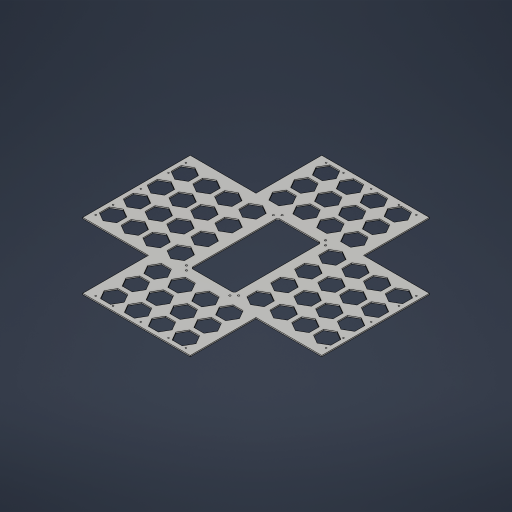
# Autodesk Inventor part: 200510
Saved by Autodesk Inventor 2023 (Build 270158000, 158)
## iProperties
Created: 2022-08-10
Part Number: 200510
Material: Aluminum 5052 H32
Document SubType Name: Sheet Metal
Designer: robotics
Density: 2.7 g/cm^3
Sheet Metal Rule: .125 5052
Appearance: Aluminum - Flat
Mass: 1564.52 g
Surface Area: 4087.8 cm^2
Volume: 579.451 cm^3
Description: Baseplate with concept geometry for pdp riser
GlobalPropertyList: <PropertyList/>
DocNumber: 200510updated.ipt
Folder: .
VDS_Category: CAD
Author: robotics
Autodesk Inventor part; units mm, degrees
ref_plane "YZ Plane" through (0, 0, 0) normal (1, 0, 0) x (0, 1, 0)
ref_plane "XZ Plane" through (0, 0, 0) normal (0, 1, 0) x (-1, 0, 0)
ref_plane "XY Plane" through (0, 0, 0) normal (0, 0, 1) x (1, 0, 0)
sketch "Sketch1" plane through (0, 0, 0) normal (0, 1, 0) x (-1, 0, 0)
  line L0 (0, 0) -> (0, -314.325)
  line L1 (0, -314.325) -> (192.0875, -314.325)
  line L2 (192.0875, -314.325) -> (192.0875, -506.4125)
  line L3 (192.0875, -506.4125) -> (506.4125, -506.4125)
  line L4 (506.4125, -506.4125) -> (506.4125, -314.325)
  line L5 (506.4125, -314.325) -> (698.5, -314.325)
  line L6 (698.5, -314.325) -> (698.5, 0)
  line L7 (698.5, 0) -> (506.4125, 0)
  line L8 (506.4125, 0) -> (506.4125, 192.0875)
  line L9 (506.4125, 192.0875) -> (192.0875, 192.0875)
  line L10 (192.0875, 192.0875) -> (192.0875, 0)
  line L11 (192.0875, 0) -> (0, 0)
  line L12 (698.5, 192.0875) -> (0, 192.0875) construction
  line L13 (0, 192.0875) -> (0, -506.4125) construction
  line L14 (0, -506.4125) -> (698.5, -506.4125) construction
  line L15 (698.5, -506.4125) -> (698.5, 192.0875) construction
  line L16 (0, -157.1625) -> (698.5, -157.1625) construction
  line L17 (349.25, 192.0875) -> (349.25, -506.4125) construction
  line L18 (412.75, -284.1625) -> (285.75, -284.1625)
  line L19 (285.75, -284.1625) -> (285.75, -30.1625)
  line L20 (285.75, -30.1625) -> (412.75, -30.1625)
  line L21 (412.75, -30.1625) -> (412.75, -284.1625)
  line L22 (412.75, -284.1625) -> (285.75, -30.1625) construction
  line L23 (285.75, -284.1625) -> (412.75, -30.1625) construction
  line L24 (285.75, -30.1625) -> (273.05, -30.1625) construction
  line L25 (285.75, -30.1625) -> (285.75, -17.4625) construction
  line L26 (412.75, -30.1625) -> (425.45, -30.1625) construction
  line L27 (412.75, -30.1625) -> (412.75, -17.4625) construction
  line L28 (412.75, -284.1625) -> (425.45, -284.1625) construction
  line L29 (412.75, -284.1625) -> (412.75, -296.8625) construction
  line L30 (285.75, -284.1625) -> (273.05, -284.1625) construction
  line L31 (285.75, -284.1625) -> (285.75, -296.8625) construction
  circle A0 centre (425.45, -30.1625) radius 2.5797
  circle A1 centre (412.75, -17.4625) radius 2.5797
  circle A2 centre (285.75, -17.4625) radius 2.5797
  circle A3 centre (273.05, -30.1625) radius 2.5797
  circle A4 centre (273.05, -284.1625) radius 2.5797
  circle A5 centre (285.75, -296.8625) radius 2.5797
  circle A6 centre (412.75, -296.8625) radius 2.5797
  circle A7 centre (425.45, -284.1625) radius 2.5797
  line L32 (213.5581, 153.9875) -> (228.2228, 179.3875)
  line L33 (228.2228, 179.3875) -> (257.5522, 179.3875)
  line L34 (257.5522, 179.3875) -> (272.2169, 153.9875)
  line L35 (272.2169, 153.9875) -> (257.5522, 128.5875)
  line L36 (257.5522, 128.5875) -> (228.2228, 128.5875)
  line L37 (228.2228, 128.5875) -> (213.5581, 153.9875)
  line L38 (298.0728, 179.3875) -> (327.4022, 179.3875)
  line L39 (283.4081, 153.9875) -> (298.0728, 179.3875)
  line L40 (298.0728, 128.5875) -> (283.4081, 153.9875)
  line L41 (327.4022, 128.5875) -> (298.0728, 128.5875)
  line L42 (342.0669, 153.9875) -> (327.4022, 128.5875)
  line L43 (327.4022, 179.3875) -> (342.0669, 153.9875)
  line L44 (367.9228, 179.3875) -> (397.2522, 179.3875)
  line L45 (353.2581, 153.9875) -> (367.9228, 179.3875)
  line L46 (367.9228, 128.5875) -> (353.2581, 153.9875)
  line L47 (397.2522, 128.5875) -> (367.9228, 128.5875)
  line L48 (411.9169, 153.9875) -> (397.2522, 128.5875)
  line L49 (397.2522, 179.3875) -> (411.9169, 153.9875)
  line L50 (437.7728, 179.3875) -> (467.1022, 179.3875)
  line L51 (423.1081, 153.9875) -> (437.7728, 179.3875)
  line L52 (437.7728, 128.5875) -> (423.1081, 153.9875)
  line L53 (467.1022, 128.5875) -> (437.7728, 128.5875)
  line L54 (481.7669, 153.9875) -> (467.1022, 128.5875)
  line L55 (467.1022, 179.3875) -> (481.7669, 153.9875)
  line L56 (228.2228, 115.8875) -> (257.5522, 115.8875)
  line L57 (213.5581, 90.4875) -> (228.2228, 115.8875)
  line L58 (228.2228, 65.0875) -> (213.5581, 90.4875)
  line L59 (257.5522, 65.0875) -> (228.2228, 65.0875)
  line L60 (272.2169, 90.4875) -> (257.5522, 65.0875)
  line L61 (257.5522, 115.8875) -> (272.2169, 90.4875)
  line L62 (298.0728, 115.8875) -> (327.4022, 115.8875)
  line L63 (283.4081, 90.4875) -> (298.0728, 115.8875)
  line L64 (298.0728, 65.0875) -> (283.4081, 90.4875)
  line L65 (327.4022, 65.0875) -> (298.0728, 65.0875)
  line L66 (342.0669, 90.4875) -> (327.4022, 65.0875)
  line L67 (327.4022, 115.8875) -> (342.0669, 90.4875)
  line L68 (367.9228, 115.8875) -> (397.2522, 115.8875)
  line L69 (353.2581, 90.4875) -> (367.9228, 115.8875)
  line L70 (367.9228, 65.0875) -> (353.2581, 90.4875)
  line L71 (397.2522, 65.0875) -> (367.9228, 65.0875)
  line L72 (411.9169, 90.4875) -> (397.2522, 65.0875)
  line L73 (397.2522, 115.8875) -> (411.9169, 90.4875)
  line L74 (437.7728, 115.8875) -> (467.1022, 115.8875)
  line L75 (423.1081, 90.4875) -> (437.7728, 115.8875)
  line L76 (437.7728, 65.0875) -> (423.1081, 90.4875)
  line L77 (467.1022, 65.0875) -> (437.7728, 65.0875)
  line L78 (481.7669, 90.4875) -> (467.1022, 65.0875)
  line L79 (467.1022, 115.8875) -> (481.7669, 90.4875)
  line L80 (228.2228, 52.3875) -> (257.5522, 52.3875)
  line L81 (213.5581, 26.9875) -> (228.2228, 52.3875)
  line L82 (228.2228, 1.5875) -> (213.5581, 26.9875)
  line L83 (257.5522, 1.5875) -> (228.2228, 1.5875)
  line L84 (272.2169, 26.9875) -> (257.5522, 1.5875)
  line L85 (257.5522, 52.3875) -> (272.2169, 26.9875)
  line L86 (298.0728, 52.3875) -> (327.4022, 52.3875)
  line L87 (283.4081, 26.9875) -> (298.0728, 52.3875)
  line L88 (298.0728, 1.5875) -> (283.4081, 26.9875)
  line L89 (327.4022, 1.5875) -> (298.0728, 1.5875)
  line L90 (342.0669, 26.9875) -> (327.4022, 1.5875)
  line L91 (327.4022, 52.3875) -> (342.0669, 26.9875)
  line L92 (367.9228, 52.3875) -> (397.2522, 52.3875)
  line L93 (353.2581, 26.9875) -> (367.9228, 52.3875)
  line L94 (367.9228, 1.5875) -> (353.2581, 26.9875)
  line L95 (397.2522, 1.5875) -> (367.9228, 1.5875)
  line L96 (411.9169, 26.9875) -> (397.2522, 1.5875)
  line L97 (397.2522, 52.3875) -> (411.9169, 26.9875)
  line L98 (437.7728, 52.3875) -> (467.1022, 52.3875)
  line L99 (423.1081, 26.9875) -> (437.7728, 52.3875)
  line L100 (437.7728, 1.5875) -> (423.1081, 26.9875)
  line L101 (467.1022, 1.5875) -> (437.7728, 1.5875)
  line L102 (481.7669, 26.9875) -> (467.1022, 1.5875)
  line L103 (467.1022, 52.3875) -> (481.7669, 26.9875)
  line L104 (38.1, -292.8544) -> (12.7, -278.1897)
  line L105 (12.7, -278.1897) -> (12.7, -248.8603)
  line L106 (12.7, -248.8603) -> (38.1, -234.1956)
  line L107 (38.1, -234.1956) -> (63.5, -248.8603)
  line L108 (127, -278.1897) -> (101.6, -292.8544)
  line L109 (101.6, -234.1956) -> (127, -248.8603)
  line L110 (76.2, -248.8603) -> (101.6, -234.1956)
  line L111 (76.2, -278.1897) -> (76.2, -248.8603)
  line L112 (101.6, -292.8544) -> (76.2, -278.1897)
  line L113 (63.5, -248.8603) -> (63.5, -278.1897)
  line L114 (63.5, -278.1897) -> (38.1, -292.8544)
  line L115 (127, -248.8603) -> (127, -278.1897)
  line L116 (12.7, -208.3397) -> (12.7, -179.0103)
  line L117 (127, -208.3397) -> (101.6, -223.0044)
  line L118 (12.7, -138.4897) -> (12.7, -109.1603)
  line L119 (101.6, -223.0044) -> (76.2, -208.3397)
  line L120 (76.2, -208.3397) -> (76.2, -179.0103)
  line L121 (63.5, -138.4897) -> (38.1, -153.1544)
  line L122 (38.1, -153.1544) -> (12.7, -138.4897)
  line L123 (38.1, -164.3456) -> (63.5, -179.0103)
  line L124 (63.5, -179.0103) -> (63.5, -208.3397)
  line L125 (63.5, -208.3397) -> (38.1, -223.0044)
  line L126 (12.7, -179.0103) -> (38.1, -164.3456)
  line L127 (38.1, -223.0044) -> (12.7, -208.3397)
  line L128 (38.1, -94.4956) -> (63.5, -109.1603)
  line L129 (12.7, -109.1603) -> (38.1, -94.4956)
  line L130 (63.5, -39.3103) -> (63.5, -68.6397)
  line L131 (38.1, -24.6456) -> (63.5, -39.3103)
  line L132 (63.5, -68.6397) -> (38.1, -83.3044)
  line L133 (12.7, -39.3103) -> (38.1, -24.6456)
  line L134 (12.7, -68.6397) -> (12.7, -39.3103)
  line L135 (38.1, -83.3044) -> (12.7, -68.6397)
  line L136 (76.2, -179.0103) -> (101.6, -164.3456)
  line L137 (101.6, -164.3456) -> (127, -179.0103)
  line L138 (63.5, -109.1603) -> (63.5, -138.4897)
  line L139 (101.6, -153.1544) -> (76.2, -138.4897)
  line L140 (76.2, -138.4897) -> (76.2, -109.1603)
  line L141 (127, -138.4897) -> (101.6, -153.1544)
  line L142 (76.2, -68.6397) -> (76.2, -39.3103)
  line L143 (76.2, -109.1603) -> (101.6, -94.4956)
  line L144 (101.6, -83.3044) -> (76.2, -68.6397)
  line L145 (101.6, -94.4956) -> (127, -109.1603)
  line L146 (127, -68.6397) -> (101.6, -83.3044)
  line L147 (76.2, -39.3103) -> (101.6, -24.6456)
  line L148 (127, -39.3103) -> (127, -68.6397)
  line L149 (101.6, -24.6456) -> (127, -39.3103)
  line L150 (139.7, -278.1897) -> (139.7, -248.8603)
  line L151 (165.1, -292.8544) -> (139.7, -278.1897)
  line L152 (139.7, -248.8603) -> (165.1, -234.1956)
  line L153 (165.1, -223.0044) -> (139.7, -208.3397)
  line L154 (190.5, -278.1897) -> (165.1, -292.8544)
  line L155 (190.5, -248.8603) -> (190.5, -278.1897)
  line L156 (165.1, -234.1956) -> (190.5, -248.8603)
  line L157 (190.5, -208.3397) -> (165.1, -223.0044)
  line L158 (127, -179.0103) -> (127, -208.3397)
  line L159 (139.7, -208.3397) -> (139.7, -179.0103)
  line L160 (190.5, -179.0103) -> (190.5, -208.3397)
  line L161 (127, -109.1603) -> (127, -138.4897)
  line L162 (165.1, -153.1544) -> (139.7, -138.4897)
  line L163 (165.1, -164.3456) -> (190.5, -179.0103)
  line L164 (139.7, -138.4897) -> (139.7, -109.1603)
  line L165 (190.5, -138.4897) -> (165.1, -153.1544)
  line L166 (190.5, -109.1603) -> (190.5, -138.4897)
  line L167 (139.7, -179.0103) -> (165.1, -164.3456)
  line L168 (165.1, -94.4956) -> (190.5, -109.1603)
  line L169 (139.7, -109.1603) -> (165.1, -94.4956)
  line L170 (190.5, -68.6397) -> (165.1, -83.3044)
  line L171 (190.5, -39.3103) -> (190.5, -68.6397)
  line L172 (139.7, -68.6397) -> (139.7, -39.3103)
  line L173 (165.1, -24.6456) -> (190.5, -39.3103)
  line L174 (139.7, -39.3103) -> (165.1, -24.6456)
  line L175 (165.1, -83.3044) -> (139.7, -68.6397)
  line L176 (484.9419, -468.3125) -> (470.2772, -493.7125)
  line L177 (470.2772, -493.7125) -> (440.9478, -493.7125)
  line L178 (440.9478, -493.7125) -> (426.2831, -468.3125)
  line L179 (426.2831, -468.3125) -> (440.9478, -442.9125)
  line L180 (470.2772, -379.4125) -> (484.9419, -404.8125)
  line L181 (426.2831, -404.8125) -> (440.9478, -379.4125)
  line L182 (440.9478, -430.2125) -> (426.2831, -404.8125)
  line L183 (470.2772, -430.2125) -> (440.9478, -430.2125)
  line L184 (484.9419, -404.8125) -> (470.2772, -430.2125)
  line L185 (440.9478, -442.9125) -> (470.2772, -442.9125)
  line L186 (470.2772, -442.9125) -> (484.9419, -468.3125)
  line L187 (440.9478, -379.4125) -> (470.2772, -379.4125)
  line L188 (400.4272, -493.7125) -> (371.0978, -493.7125)
  line L189 (400.4272, -379.4125) -> (415.0919, -404.8125)
  line L190 (330.5772, -493.7125) -> (301.2478, -493.7125)
  line L191 (415.0919, -404.8125) -> (400.4272, -430.2125)
  line L192 (400.4272, -430.2125) -> (371.0978, -430.2125)
  line L193 (330.5772, -442.9125) -> (345.2419, -468.3125)
  line L194 (345.2419, -468.3125) -> (330.5772, -493.7125)
  line L195 (356.4331, -468.3125) -> (371.0978, -442.9125)
  line L196 (371.0978, -442.9125) -> (400.4272, -442.9125)
  line L197 (400.4272, -442.9125) -> (415.0919, -468.3125)
  line L198 (371.0978, -493.7125) -> (356.4331, -468.3125)
  line L199 (415.0919, -468.3125) -> (400.4272, -493.7125)
  line L200 (286.5831, -468.3125) -> (301.2478, -442.9125)
  line L201 (301.2478, -493.7125) -> (286.5831, -468.3125)
  line L202 (231.3978, -442.9125) -> (260.7272, -442.9125)
  line L203 (216.7331, -468.3125) -> (231.3978, -442.9125)
  line L204 (260.7272, -442.9125) -> (275.3919, -468.3125)
  line L205 (231.3978, -493.7125) -> (216.7331, -468.3125)
  line L206 (260.7272, -493.7125) -> (231.3978, -493.7125)
  line L207 (275.3919, -468.3125) -> (260.7272, -493.7125)
  line L208 (371.0978, -430.2125) -> (356.4331, -404.8125)
  line L209 (356.4331, -404.8125) -> (371.0978, -379.4125)
  line L210 (301.2478, -442.9125) -> (330.5772, -442.9125)
  line L211 (345.2419, -404.8125) -> (330.5772, -430.2125)
  line L212 (330.5772, -430.2125) -> (301.2478, -430.2125)
  line L213 (330.5772, -379.4125) -> (345.2419, -404.8125)
  line L214 (260.7272, -430.2125) -> (231.3978, -430.2125)
  line L215 (301.2478, -430.2125) -> (286.5831, -404.8125)
  line L216 (275.3919, -404.8125) -> (260.7272, -430.2125)
  line L217 (286.5831, -404.8125) -> (301.2478, -379.4125)
  line L218 (260.7272, -379.4125) -> (275.3919, -404.8125)
  line L219 (231.3978, -430.2125) -> (216.7331, -404.8125)
  line L220 (231.3978, -379.4125) -> (260.7272, -379.4125)
  line L221 (216.7331, -404.8125) -> (231.3978, -379.4125)
  line L222 (470.2772, -366.7125) -> (440.9478, -366.7125)
  line L223 (484.9419, -341.3125) -> (470.2772, -366.7125)
  line L224 (440.9478, -366.7125) -> (426.2831, -341.3125)
  line L225 (415.0919, -341.3125) -> (400.4272, -366.7125)
  line L226 (470.2772, -315.9125) -> (484.9419, -341.3125)
  line L227 (440.9478, -315.9125) -> (470.2772, -315.9125)
  line L228 (426.2831, -341.3125) -> (440.9478, -315.9125)
  line L229 (400.4272, -315.9125) -> (415.0919, -341.3125)
  line L230 (371.0978, -379.4125) -> (400.4272, -379.4125)
  line L231 (400.4272, -366.7125) -> (371.0978, -366.7125)
  line L232 (371.0978, -315.9125) -> (400.4272, -315.9125)
  line L233 (301.2478, -379.4125) -> (330.5772, -379.4125)
  line L234 (345.2419, -341.3125) -> (330.5772, -366.7125)
  line L235 (356.4331, -341.3125) -> (371.0978, -315.9125)
  line L236 (330.5772, -366.7125) -> (301.2478, -366.7125)
  line L237 (330.5772, -315.9125) -> (345.2419, -341.3125)
  line L238 (301.2478, -315.9125) -> (330.5772, -315.9125)
  line L239 (371.0978, -366.7125) -> (356.4331, -341.3125)
  line L240 (286.5831, -341.3125) -> (301.2478, -315.9125)
  line L241 (301.2478, -366.7125) -> (286.5831, -341.3125)
  line L242 (260.7272, -315.9125) -> (275.3919, -341.3125)
  line L243 (231.3978, -315.9125) -> (260.7272, -315.9125)
  line L244 (260.7272, -366.7125) -> (231.3978, -366.7125)
  line L245 (216.7331, -341.3125) -> (231.3978, -315.9125)
  line L246 (231.3978, -366.7125) -> (216.7331, -341.3125)
  line L247 (275.3919, -341.3125) -> (260.7272, -366.7125)
  line L248 (660.4, -21.4706) -> (685.8, -36.1353)
  line L249 (685.8, -36.1353) -> (685.8, -65.4647)
  line L250 (685.8, -65.4647) -> (660.4, -80.1294)
  line L251 (660.4, -80.1294) -> (635, -65.4647)
  line L252 (571.5, -36.1353) -> (596.9, -21.4706)
  line L253 (596.9, -80.1294) -> (571.5, -65.4647)
  line L254 (622.3, -65.4647) -> (596.9, -80.1294)
  line L255 (622.3, -36.1353) -> (622.3, -65.4647)
  line L256 (596.9, -21.4706) -> (622.3, -36.1353)
  line L257 (635, -65.4647) -> (635, -36.1353)
  line L258 (635, -36.1353) -> (660.4, -21.4706)
  line L259 (571.5, -65.4647) -> (571.5, -36.1353)
  line L260 (685.8, -105.9853) -> (685.8, -135.3147)
  line L261 (571.5, -105.9853) -> (596.9, -91.3206)
  line L262 (685.8, -175.8353) -> (685.8, -205.1647)
  line L263 (596.9, -91.3206) -> (622.3, -105.9853)
  line L264 (622.3, -105.9853) -> (622.3, -135.3147)
  line L265 (635, -175.8353) -> (660.4, -161.1706)
  line L266 (660.4, -161.1706) -> (685.8, -175.8353)
  line L267 (660.4, -149.9794) -> (635, -135.3147)
  line L268 (635, -135.3147) -> (635, -105.9853)
  line L269 (635, -105.9853) -> (660.4, -91.3206)
  line L270 (685.8, -135.3147) -> (660.4, -149.9794)
  line L271 (660.4, -91.3206) -> (685.8, -105.9853)
  line L272 (660.4, -219.8294) -> (635, -205.1647)
  line L273 (685.8, -205.1647) -> (660.4, -219.8294)
  line L274 (635, -275.0147) -> (635, -245.6853)
  line L275 (660.4, -289.6794) -> (635, -275.0147)
  line L276 (635, -245.6853) -> (660.4, -231.0206)
  line L277 (685.8, -275.0147) -> (660.4, -289.6794)
  line L278 (685.8, -245.6853) -> (685.8, -275.0147)
  line L279 (660.4, -231.0206) -> (685.8, -245.6853)
  line L280 (622.3, -135.3147) -> (596.9, -149.9794)
  line L281 (596.9, -149.9794) -> (571.5, -135.3147)
  line L282 (635, -205.1647) -> (635, -175.8353)
  line L283 (596.9, -161.1706) -> (622.3, -175.8353)
  line L284 (622.3, -175.8353) -> (622.3, -205.1647)
  line L285 (571.5, -175.8353) -> (596.9, -161.1706)
  line L286 (622.3, -245.6853) -> (622.3, -275.0147)
  line L287 (622.3, -205.1647) -> (596.9, -219.8294)
  line L288 (596.9, -231.0206) -> (622.3, -245.6853)
  line L289 (596.9, -219.8294) -> (571.5, -205.1647)
  line L290 (571.5, -245.6853) -> (596.9, -231.0206)
  line L291 (622.3, -275.0147) -> (596.9, -289.6794)
  line L292 (571.5, -275.0147) -> (571.5, -245.6853)
  line L293 (596.9, -289.6794) -> (571.5, -275.0147)
  line L294 (558.8, -36.1353) -> (558.8, -65.4647)
  line L295 (533.4, -21.4706) -> (558.8, -36.1353)
  line L296 (558.8, -65.4647) -> (533.4, -80.1294)
  line L297 (533.4, -91.3206) -> (558.8, -105.9853)
  line L298 (508, -36.1353) -> (533.4, -21.4706)
  line L299 (508, -65.4647) -> (508, -36.1353)
  line L300 (533.4, -80.1294) -> (508, -65.4647)
  line L301 (508, -105.9853) -> (533.4, -91.3206)
  line L302 (571.5, -135.3147) -> (571.5, -105.9853)
  line L303 (558.8, -105.9853) -> (558.8, -135.3147)
  line L304 (508, -135.3147) -> (508, -105.9853)
  line L305 (571.5, -205.1647) -> (571.5, -175.8353)
  line L306 (533.4, -161.1706) -> (558.8, -175.8353)
  line L307 (533.4, -149.9794) -> (508, -135.3147)
  line L308 (558.8, -175.8353) -> (558.8, -205.1647)
  line L309 (508, -175.8353) -> (533.4, -161.1706)
  line L310 (508, -205.1647) -> (508, -175.8353)
  line L311 (558.8, -135.3147) -> (533.4, -149.9794)
  line L312 (533.4, -219.8294) -> (508, -205.1647)
  line L313 (558.8, -205.1647) -> (533.4, -219.8294)
  line L314 (508, -245.6853) -> (533.4, -231.0206)
  line L315 (508, -275.0147) -> (508, -245.6853)
  line L316 (558.8, -245.6853) -> (558.8, -275.0147)
  line L317 (533.4, -289.6794) -> (508, -275.0147)
  line L318 (558.8, -275.0147) -> (533.4, -289.6794)
  line L319 (533.4, -231.0206) -> (558.8, -245.6853)
  line L320 (258.0906, -39.3103) -> (258.0906, -68.6397)
  line L321 (258.0906, -68.6397) -> (232.6906, -83.3044)
  line L322 (232.6906, -83.3044) -> (207.2906, -68.6397)
  line L323 (207.2906, -68.6397) -> (207.2906, -39.3103)
  line L324 (207.2906, -39.3103) -> (232.6906, -24.6456)
  line L325 (232.6906, -24.6456) -> (258.0906, -39.3103)
  line L326 (232.6906, -153.1544) -> (207.2906, -138.4897)
  line L327 (207.2906, -138.4897) -> (207.2906, -109.1603)
  line L328 (207.2906, -109.1603) -> (232.6906, -94.4956)
  line L329 (232.6906, -94.4956) -> (258.0906, -109.1603)
  line L330 (258.0906, -109.1603) -> (258.0906, -138.4897)
  line L331 (258.0906, -138.4897) -> (232.6906, -153.1544)
  line L332 (232.6906, -223.0044) -> (207.2906, -208.3397)
  line L333 (207.2906, -208.3397) -> (207.2906, -179.0103)
  line L334 (207.2906, -179.0103) -> (232.6906, -164.3456)
  line L335 (232.6906, -164.3456) -> (258.0906, -179.0103)
  line L336 (258.0906, -179.0103) -> (258.0906, -208.3397)
  line L337 (258.0906, -208.3397) -> (232.6906, -223.0044)
  line L338 (232.6906, -292.8544) -> (207.2906, -278.1897)
  line L339 (207.2906, -278.1897) -> (207.2906, -248.8603)
  line L340 (207.2906, -248.8603) -> (232.6906, -234.1956)
  line L341 (232.6906, -234.1956) -> (258.0906, -248.8603)
  line L342 (258.0906, -248.8603) -> (258.0906, -278.1897)
  line L343 (258.0906, -278.1897) -> (232.6906, -292.8544)
  line L344 (440.4094, -39.3103) -> (440.4094, -68.6397)
  line L345 (440.4094, -68.6397) -> (465.8094, -83.3044)
  line L346 (465.8094, -83.3044) -> (491.2094, -68.6397)
  line L347 (491.2094, -68.6397) -> (491.2094, -39.3103)
  line L348 (491.2094, -39.3103) -> (465.8094, -24.6456)
  line L349 (465.8094, -24.6456) -> (440.4094, -39.3103)
  line L350 (465.8094, -153.1544) -> (491.2094, -138.4897)
  line L351 (491.2094, -138.4897) -> (491.2094, -109.1603)
  line L352 (491.2094, -109.1603) -> (465.8094, -94.4956)
  line L353 (465.8094, -94.4956) -> (440.4094, -109.1603)
  line L354 (440.4094, -109.1603) -> (440.4094, -138.4897)
  line L355 (440.4094, -138.4897) -> (465.8094, -153.1544)
  line L356 (465.8094, -223.0044) -> (491.2094, -208.3397)
  line L357 (491.2094, -208.3397) -> (491.2094, -179.0103)
  line L358 (491.2094, -179.0103) -> (465.8094, -164.3456)
  line L359 (465.8094, -164.3456) -> (440.4094, -179.0103)
  line L360 (440.4094, -179.0103) -> (440.4094, -208.3397)
  line L361 (440.4094, -208.3397) -> (465.8094, -223.0044)
  line L362 (465.8094, -292.8544) -> (491.2094, -278.1897)
  line L363 (491.2094, -278.1897) -> (491.2094, -248.8603)
  line L364 (491.2094, -248.8603) -> (465.8094, -234.1956)
  line L365 (465.8094, -234.1956) -> (440.4094, -248.8603)
  line L366 (440.4094, -248.8603) -> (440.4094, -278.1897)
  line L367 (440.4094, -278.1897) -> (465.8094, -292.8544)
  point P0 (349.25, -157.1625)
  point P1 (242.8875, 153.9875)
  point P2 (312.7375, 153.9875)
  point P3 (382.5875, 153.9875)
  point P4 (452.4375, 153.9875)
  point P5 (242.8875, 90.4875)
  point P6 (312.7375, 90.4875)
  point P7 (382.5875, 90.4875)
  point P8 (452.4375, 90.4875)
  point P9 (242.8875, 26.9875)
  point P10 (312.7375, 26.9875)
  point P11 (382.5875, 26.9875)
  point P12 (452.4375, 26.9875)
  point P13 (38.1, -263.525)
  point P14 (101.6, -263.525)
  point P15 (101.6, -193.675)
  point P16 (38.1, -193.675)
  point P17 (38.1, -53.975)
  point P18 (38.1, -123.825)
  point P19 (101.6, -123.825)
  point P20 (101.6, -53.975)
  point P21 (165.1, -263.525)
  point P22 (165.1, -193.675)
  point P23 (165.1, -123.825)
  point P24 (165.1, -53.975)
  point P25 (455.6125, -468.3125)
  point P26 (455.6125, -404.8125)
  point P27 (385.7625, -404.8125)
  point P28 (385.7625, -468.3125)
  point P29 (246.0625, -468.3125)
  point P30 (315.9125, -468.3125)
  point P31 (315.9125, -404.8125)
  point P32 (246.0625, -404.8125)
  point P33 (455.6125, -341.3125)
  point P34 (385.7625, -341.3125)
  point P35 (315.9125, -341.3125)
  point P36 (246.0625, -341.3125)
  point P37 (660.4, -50.8)
  point P38 (596.9, -50.8)
  point P39 (596.9, -120.65)
  point P40 (660.4, -120.65)
  point P41 (660.4, -260.35)
  point P42 (660.4, -190.5)
  point P43 (596.9, -190.5)
  point P44 (596.9, -260.35)
  point P45 (533.4, -50.8)
  point P46 (533.4, -120.65)
  point P47 (533.4, -190.5)
  point P48 (533.4, -260.35)
  point P49 (232.6906, -53.975)
  point P50 (232.6906, -123.825)
  point P51 (232.6906, -193.675)
  point P52 (232.6906, -263.525)
  point P53 (465.8094, -53.975)
  point P54 (465.8094, -123.825)
  point P55 (465.8094, -193.675)
  point P56 (465.8094, -263.525)
  dimension "d0" = 698.5
  dimension "d1" = 192.0875
  dimension "d43" = 127
  dimension "d44" = 254
  dimension "d46" = 12.7
  dimension "d47" = 12.7
  dimension "d48" = 12.7
  dimension "d49" = 12.7
  dimension "d50" = 12.7
  dimension "d51" = 12.7
  dimension "d52" = 12.7
  dimension "d53" = 12.7
  dimension "d54" = 5.1594
  dimension "d55" = 25.4
  dimension "d56" = 38.1
  dimension "d57" = 50.8
  dimension "d60" = 69.85
  dimension "d63" = 63.5
  dimension "d68" = 360
  dimension "d72" = 69.85
  dimension "d77" = 16.7906
  measures "d0" distance of L14.end L12.start
  measures "d1" distance of L7.end L8.end
  measures "d43" distance of L19.end L20.end
  measures "d44" distance of L18.end L19.end
  measures "d46" distance of L19.end L24.end
  measures "d47" distance of L19.end L25.end
  measures "d48" distance of L20.end L26.end
  measures "d49" distance of L20.end L27.end
  measures "d50" distance of L18.start L28.end
  measures "d51" distance of L18.start L29.end
  measures "d52" distance of L18.end L30.end
  measures "d53" distance of L18.end L31.end
  measures "d54" diameter of A0
  measures "d55" vertical distance of L33.end L34.end
  measures "d56" distance from line of L9 point (242.887, 153.988)
  measures "d57" distance from line of L10 point (242.887, 153.988)
  measures "d60" distance of L32.end L38.start
  measures "d63" distance of L32.end L56.start
  measures "d72" distance of point (232.691, -53.975) point (232.691, -123.825)
  measures "d77" distance between parallel lines of L171 L323
extrude "Plate1" add sketch "Sketch1" along normal blind 3.175
sketch "Sketch2" plane through (0, 3.175, 0) normal (0, 1, 0) x (1, 0, 0)
  line L0 (-506.4125, 506.4125) -> (-192.0875, 506.4125) projected
  line L1 (0, 314.325) -> (0, 0) projected
  line L2 (-192.0875, -192.0875) -> (-506.4125, -192.0875) projected
  line L3 (-698.5, 0) -> (-698.5, 314.325) projected
  line L4 (-506.4125, 314.325) -> (-506.4125, 506.4125) projected
  line L5 (-192.0875, 506.4125) -> (-192.0875, 314.325) projected
  line L6 (-698.5, 314.325) -> (-506.4125, 314.325) projected
  line L7 (-506.4125, 0) -> (-698.5, 0) projected
  line L8 (-349.25, 506.4125) -> (-349.25, -192.0875) construction
  line L9 (-698.5, 157.1625) -> (0, 157.1625) construction
  point P0 (-481.0125, 493.7125)
  point P1 (-430.2125, 493.7125)
  point P2 (-268.2875, 493.7125)
  point P3 (-217.4875, 493.7125)
  point P4 (-12.7, 288.925)
  point P5 (-12.7, 238.125)
  point P6 (-12.7, 76.2)
  point P7 (-12.7, 25.4)
  point P8 (-217.4875, -179.3875)
  point P9 (-268.2875, -179.3875)
  point P10 (-430.2125, -179.3875)
  point P11 (-481.0125, -179.3875)
  point P12 (-685.8, 25.4)
  point P13 (-685.8, 76.2)
  point P14 (-685.8, 238.125)
  point P15 (-685.8, 288.925)
  point P16 (-349.25, 493.7125)
  point P17 (-349.25, -179.3875)
  point P18 (-685.8, 157.1625)
  point P19 (-12.7, 157.1625)
  dimension "d3" = 12.7
  dimension "d4" = 12.7
  dimension "d5" = 12.7
  dimension "d6" = 12.7
  dimension "d7" = 25.4
  dimension "d8" = 50.8
  dimension "d9" = 25.4
  dimension "d10" = 50.8
  dimension "d11" = 25.4
  dimension "d12" = 50.8
  dimension "d13" = 25.4
  dimension "d14" = 50.8
  constraints: 12 horizontal alignment, 12 vertical alignment, 4 end point, 4 midpoint, 4 point on line
  measures "d3" distance from line of L0 point (-481.012, 493.712)
  measures "d4" distance from line of L1 point (-12.7, 288.925)
  measures "d5" distance from line of L2 point (-217.488, -179.388)
  measures "d6" distance from line of L3 point (-685.8, 288.925)
  measures "d7" distance from line of L4 point (-481.012, 493.712)
  measures "d8" distance of point (-430.212, 493.712) point (-481.012, 493.712)
  measures "d9" distance from line of L5 point (-217.488, 493.712)
  measures "d10" distance of point (-268.288, 493.712) point (-217.488, 493.712)
  measures "d11" distance from line of L6 point (-685.8, 288.925)
  measures "d12" distance of point (-685.8, 288.925) point (-685.8, 238.125)
  measures "d13" distance from line of L7 point (-685.8, 25.4)
  measures "d14" distance of point (-685.8, 76.2) point (-685.8, 25.4)
hole "Hole1" at (-685.8, 3.175, -288.925) at (-685.8, 3.175, -238.125) at (-685.8, 3.175, -76.2) at (-685.8, 3.175, -25.4) at (-481.0125, 3.175, 179.3875) at (-430.2125, 3.175, 179.3875) at (-268.2875, 3.175, 179.3875) at (-217.4875, 3.175, 179.3875) at (-12.7, 3.175, -25.4) at (-12.7, 3.175, -76.2) at (-12.7, 3.175, -238.125) at (-12.7, 3.175, -288.925) at (-217.4875, 3.175, -493.7125) at (-268.2875, 3.175, -493.7125) at (-430.2125, 3.175, -493.7125) at (-481.0125, 3.175, -493.7125) at (-685.8, 3.175, -157.1625) at (-349.25, 3.175, 179.3875) at (-12.7, 3.175, -157.1625) at (-349.25, 3.175, -493.7125) direction (0, -1, 0) diameter 4.0894 end through all clearance for "Pop Rivet" size "5/32" standard "4859 Fastners"
sketch "Sketch3" plane through (0, 3.175, 0) normal (0, 1, 0) x (1, 0, 0)
  circle A0 centre (-12.7, 25.4) radius 2.0447 construction
sketch "Sketch4" plane through (0, 3.175, 0) normal (0, 1, 0) x (1, 0, 0)
  circle A0 centre (-12.7, 76.2) radius 2.0447 construction
fillet "Corner Round1" radius 6.35 4 edges at (-412.75, 1.5875, -284.1625) (-285.75, 1.5875, -284.1625) (-412.75, 1.5875, -30.1625) (-285.75, 1.5875, -30.1625)
equation "\"d9\" = d7"
equation "\"d10\" = d8"
equation "\"d11\" = d7"
equation "\"d12\" = d8"
equation "\"d13\" = d7"
equation "\"d14\" = d8"
equation "\"d0\" = DrivebaseLength"
equation "\"d1\" = PlateCut"
equation "\"d20\" = Thickness"
equation "\"d2\" = Thickness"
equation "\"BendRadius\" = 1.5 * Thickness"
equation "\"BendReliefWidth\" = Thickness"
equation "\"BendReliefDepth\" = 0.5 * Thickness"
equation "\"CornerReliefSize\" = 4 * Thickness"
equation "\"MinimumRemnant\" = 2 * Thickness"
equation "\"TransitionRadius\" = BendRadius"
equation "\"JacobiRadiusSize\" = BendRadius"
equation "\"GapSize\" = Thickness"
equation "\"DrivebaseLength\" = 698.5"
equation "\"DrivebaseWidth\" = 698.5"
equation "\"LengthOfTube\" = 482.6"
equation "\"ModuleSize\" = 169.8625"
equation "\"EdgeModuleToHole\" = 61.9125"
equation "\"ModuleSpace\" = 107.95"
equation "\"HoleLength1\" = 6.35"
equation "\"HoleLength2\" = 31.75"
equation "\"HoleLength3\" = 57.15"
equation "\"HoleLength4\" = 425.45"
equation "\"HoleLength5\" = 450.85"
equation "\"HoleLength6\" = 476.25"
equation "\"HoleWidth\" = 12.7"
equation "\"ModuleLength\" = 190.5"
equation "\"PlateCut\" = 192.0875"
equation "\"Rivet1\" = 109.5375"
equation "\"Rivet2\" = 160.3375"
equation "\"Rivet4\" = 322.2625"
equation "\"Rivet3\" = 241.3"
equation "\"Rivet5\" = 373.0625"
equation "\"Thickness\" = 3.175"
body "Solid1"
